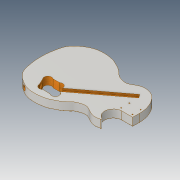
# Autodesk Inventor part: Corpo2
Saved by Autodesk Inventor 2016 (Build 200138000, 138)
## iProperties
Created: 2018-10-15
Part Number: Corpo2
Material: Generic
Document SubType Name: Modeling
Designer: Pedro Mendonça
Density: 1 g/cm^3
Appearance: Yellow Pine - Solid Stained Light Low Gloss
Author: Pedro Mendonça
Autodesk Inventor part; units mm, degrees
ref_plane "YZ Plane" through (0, 0, 0) normal (1, 0, 0) x (0, 1, 0)
ref_plane "XZ Plane" through (0, 0, 0) normal (0, 1, 0) x (-1, 0, 0)
ref_plane "XY Plane" through (0, 0, 0) normal (0, 0, 1) x (1, 0, 0)
sketch "Sketch1" plane through (0, 0, 0) normal (0, 0, 1) x (1, 0, 0)
  line L0 (0, 0) -> (0, -455) construction
  line L1 (0, -153) -> (-92, -153) construction
  line L2 (0, -435) -> (-103, -435) construction
  line L3 (0, -415) -> (-122, -415) construction
  line L4 (-0.0087, -394.9827) -> (-140.0087, -394.9827) construction
  line L5 (0, -375) -> (-151, -375) construction
  line L6 (0, -355) -> (-158, -355) construction
  line L7 (0, -335) -> (-160, -335) construction
  line L8 (0, -315) -> (-161, -315) construction
  line L9 (0, -295) -> (-158, -295) construction
  line L10 (0, -275) -> (-154, -275) construction
  line L11 (0, -255) -> (-145, -255) construction
  line L12 (0, -235) -> (-135, -235) construction
  line L13 (0, -215) -> (-120, -215) construction
  line L14 (0, -195) -> (-103, -195) construction
  line L15 (0, -175) -> (-95, -175) construction
  line L16 (0, -135) -> (-98, -135) construction
  line L17 (0, -115) -> (-109, -115) construction
  line L18 (0, -95) -> (-115, -95) construction
  line L19 (0, -75) -> (-114, -75) construction
  line L20 (0, -55) -> (-108, -55) construction
  line L21 (0, -35) -> (-93.9417, -35) construction
  line L22 (0, -15) -> (-65, -15) construction
  line L23 (0, -455) -> (-21.0472, -455.5046) construction
  line L24 (-159.5472, -351.6393) -> (-160.2622, -336.1037) construction
  line L25 (-64.2186, -11.8549) -> (-30.25, 0) construction
  line L26 (-30.25, 0) -> (0, 0) construction
  spline S0 degree 4 poles (0, -455) (-21.0472, -455.5046) (-39.9161, -452.9713) (-55.0288, -449.8264) (-72.5, -447.3805) (-90.9559, -441.7244) (-101.5897, -436.4609) (-110.5874, -430.5207) (-124.2149, -416.631) (-132.7759, -406.8471) (-140.8913, -395.5086) (-146.9896, -384.4071) (-152.044, -373.8933) (-155.7121, -363.9428) (-159.5472, -351.6393) (-160.2622, -336.1037) (-161.3959, -321.0408) (-160.7041, -310.0555) (-158.9541, -299.1238) (-157.4845, -291.3466) (-155.7121, -278.8181) (-152.3095, -270.0787) (-148.4765, -261.546) (-144.1012, -253.4714) (-138.9752, -242.9989) (-135, -233.5666) (-126.4423, -222.6445) (-115.9364, -209.2361) (-106.2015, -200.3968) (-100.5222, -191.8137) (-95.3552, -177.4658) (-92.8358, -167.4735) (-90.7434, -152.656) (-94.3304, -141.7669) (-99.2411, -132.3298) (-104.9533, -123.6353) (-111.1925, -111.3398) (-114.7925, -100.8201) (-115.9364, -86.2479) (-114.1418, -74.0378) (-111.6352, -63.1761) (-106.7365, -51.5397) (-99.6977, -40.3072) (-84.235, -25) (-64.2186, -11.8549) (-30.25, 0) (0, 0) knots 1 1 1 1 1 1.192103 1.235764 1.325453 1.466485 1.477925 1.676642 2 2.143283 3 3.486615 3.82198 4 5 6 6.816415 7 7.358575 8 8.561677 9 9.306621 10 10.059652 11 11.392225 12 12.736138 13 14 14.050123 15 15.249645 16 16.147201 17 17.733562 18 19 19.360293 20 20.169025 21 22 22 22 22 22
  line L27 (-99.6977, -40.3072) -> (-84.235, -25) construction
  line L28 (-84.235, -25) -> (-64.2186, -11.8549) construction
  line L29 (-114.1418, -74.0378) -> (-111.6352, -63.1761) construction
  line L30 (-111.6352, -63.1761) -> (-106.7365, -51.5397) construction
  line L31 (-106.7365, -51.5397) -> (-99.6977, -40.3072) construction
  line L32 (-114.7925, -100.8201) -> (-115.9364, -86.2479) construction
  line L33 (-115.9364, -86.2479) -> (-114.1418, -74.0378) construction
  line L34 (-104.9533, -123.6353) -> (-111.1925, -111.3398) construction
  line L35 (-111.1925, -111.3398) -> (-114.7925, -100.8201) construction
  line L36 (-94.3304, -141.7669) -> (-99.2411, -132.3298) construction
  line L37 (-99.2411, -132.3298) -> (-104.9533, -123.6353) construction
  line L38 (-95.3552, -177.4658) -> (-92.8358, -167.4735) construction
  line L39 (-92.8358, -167.4735) -> (-90.7434, -152.656) construction
  line L40 (-90.7434, -152.656) -> (-94.3304, -141.7669) construction
  line L41 (-106.2015, -200.3968) -> (-100.5222, -191.8137) construction
  line L42 (-100.5222, -191.8137) -> (-95.3552, -177.4658) construction
  line L43 (-126.4423, -222.6445) -> (-115.9364, -209.2361) construction
  line L44 (-115.9364, -209.2361) -> (-106.2015, -200.3968) construction
  line L45 (-138.9752, -242.9989) -> (-135, -233.5666) construction
  line L46 (-135, -233.5666) -> (-126.4423, -222.6445) construction
  line L47 (-148.4765, -261.546) -> (-144.1012, -253.4714) construction
  line L48 (-144.1012, -253.4714) -> (-138.9752, -242.9989) construction
  line L49 (-155.7121, -278.8181) -> (-152.3095, -270.0787) construction
  line L50 (-152.3095, -270.0787) -> (-148.4765, -261.546) construction
  line L51 (-158.9541, -299.1238) -> (-157.4845, -291.3466) construction
  line L52 (-157.4845, -291.3466) -> (-155.7121, -278.8181) construction
  line L53 (-160.2622, -336.1037) -> (-161.3959, -321.0408) construction
  line L54 (-161.3959, -321.0408) -> (-160.7041, -310.0555) construction
  line L55 (-160.7041, -310.0555) -> (-158.9541, -299.1238) construction
  line L56 (-146.9896, -384.4071) -> (-152.044, -373.8933) construction
  line L57 (-152.044, -373.8933) -> (-155.7121, -363.9428) construction
  line L58 (-155.7121, -363.9428) -> (-159.5472, -351.6393) construction
  line L59 (-132.7759, -406.8471) -> (-140.8913, -395.5086) construction
  line L60 (-140.8913, -395.5086) -> (-146.9896, -384.4071) construction
  line L61 (-124.2149, -416.631) -> (-132.7759, -406.8471) construction
  line L62 (-110.5874, -430.5207) -> (-124.2149, -416.631) construction
  line L63 (-90.9559, -441.7244) -> (-101.5897, -436.4609) construction
  line L64 (-101.5897, -436.4609) -> (-110.5874, -430.5207) construction
  line L65 (-21.0472, -455.5046) -> (-39.9161, -452.9713) construction
  line L66 (-39.9161, -452.9713) -> (-55.0288, -449.8264) construction
  line L67 (-55.0288, -449.8264) -> (-72.5, -447.3805) construction
  line L68 (-72.5, -447.3805) -> (-90.9559, -441.7244) construction
  line L69 (0, -455) -> (21.0472, -455.5046) construction
  line L70 (159.5472, -351.6393) -> (160.2622, -336.1037) construction
  line L71 (114.7925, -100.8201) -> (115.8966, -86.7554) construction
  line L72 (104.9533, -123.6353) -> (111.1925, -111.3398) construction
  line L73 (111.1925, -111.3398) -> (114.7925, -100.8201) construction
  line L74 (94.3304, -141.7669) -> (99.2411, -132.3298) construction
  line L75 (99.2411, -132.3298) -> (104.9533, -123.6353) construction
  line L76 (95.3552, -177.4658) -> (92.8358, -167.4735) construction
  line L77 (92.8358, -167.4735) -> (90.7434, -152.656) construction
  line L78 (90.7434, -152.656) -> (94.3304, -141.7669) construction
  line L79 (106.2015, -200.3968) -> (100.5222, -191.8137) construction
  line L80 (100.5222, -191.8137) -> (95.3552, -177.4658) construction
  line L81 (126.4423, -222.6445) -> (115.9364, -209.2361) construction
  line L82 (115.9364, -209.2361) -> (106.2015, -200.3968) construction
  line L83 (138.9752, -242.9989) -> (135, -233.5666) construction
  line L84 (135, -233.5666) -> (126.4423, -222.6445) construction
  line L85 (148.4765, -261.546) -> (144.1012, -253.4714) construction
  line L86 (144.1012, -253.4714) -> (138.9752, -242.9989) construction
  line L87 (155.7121, -278.8181) -> (152.3095, -270.0787) construction
  line L88 (152.3095, -270.0787) -> (148.4765, -261.546) construction
  line L89 (158.9541, -299.1238) -> (157.4845, -291.3466) construction
  line L90 (157.4845, -291.3466) -> (155.7121, -278.8181) construction
  line L91 (160.2622, -336.1037) -> (161.3959, -321.0408) construction
  line L92 (161.3959, -321.0408) -> (160.7041, -310.0555) construction
  line L93 (160.7041, -310.0555) -> (158.9541, -299.1238) construction
  line L94 (146.9896, -384.4071) -> (152.044, -373.8933) construction
  line L95 (152.044, -373.8933) -> (155.7121, -363.9428) construction
  line L96 (155.7121, -363.9428) -> (159.5472, -351.6393) construction
  line L97 (132.7759, -406.8471) -> (140.8913, -395.5086) construction
  line L98 (140.8913, -395.5086) -> (146.9896, -384.4071) construction
  line L99 (124.2149, -416.631) -> (132.7759, -406.8471) construction
  line L100 (110.5874, -430.5207) -> (124.2149, -416.631) construction
  line L101 (90.9559, -441.7244) -> (101.5897, -436.4609) construction
  line L102 (101.5897, -436.4609) -> (110.5874, -430.5207) construction
  line L103 (21.0472, -455.5046) -> (39.9161, -452.9713) construction
  line L104 (39.9161, -452.9713) -> (55.0288, -449.8264) construction
  line L105 (55.0288, -449.8264) -> (72.5, -447.3805) construction
  line L106 (72.5, -447.3805) -> (90.9559, -441.7244) construction
  line L107 (0, 0) -> (30, 0)
  line L108 (30, 0) -> (30, -50)
  line L109 (30, -50) -> (70, -50) construction
  arc A0 (30, -50) -> (106.5425, -66.2679) centre (70, -50) ccw
  arc A1 (112.1757, -66.6921) -> (106.5425, -66.2679) centre (109.2832, -67.488) ccw
  spline S1 degree 4 poles (0, -455) (21.0472, -455.5046) (39.9161, -452.9713) (55.0288, -449.8264) (72.5, -447.3805) (90.9559, -441.7244) (101.5897, -436.4609) (110.5874, -430.5207) (124.2149, -416.631) (132.7759, -406.8471) (140.8913, -395.5086) (146.9896, -384.4071) (152.044, -373.8933) (155.7121, -363.9428) (159.5472, -351.6393) (160.2622, -336.1037) (161.3959, -321.0408) (160.7041, -310.0555) (158.9541, -299.1238) (157.4845, -291.3466) (155.7121, -278.8181) (152.3095, -270.0787) (148.4765, -261.546) (144.1012, -253.4714) (138.9752, -242.9989) (135, -233.5666) (126.4423, -222.6445) (115.9364, -209.2361) (106.2015, -200.3968) (100.5222, -191.8137) (95.3552, -177.4658) (92.8358, -167.4735) (90.7434, -152.656) (94.3304, -141.7669) (99.2411, -132.3298) (104.9533, -123.6353) (111.1925, -111.3398) (114.7925, -100.8201) (115.8966, -86.7554) (114.5611, -76.9293) (113.4123, -71.1859) (112.1752, -66.6903) knots 1 1 1 1 1 1.192103 1.235764 1.325453 1.466485 1.477925 1.676642 2 2.143283 3 3.486615 3.82198 4 5 6 6.816415 7 7.358575 8 8.561677 9 9.306621 10 10.059652 11 11.392225 12 12.736138 13 14 14.050123 15 15.249645 16 16.147201 17 17.733562 18 18.900639 18.900639 18.900639 18.900639 18.900639
  line L110 (115.8966, -86.7554) -> (114.5611, -76.9293) construction
  line L111 (114.5611, -76.9293) -> (113.4123, -71.1859) construction
  line L112 (113.4123, -71.1859) -> (112.1752, -66.6903) construction
  dimension "d85" = 30
  dimension "d87" = 90
  dimension "d88" = 40
  dimension "d95" = 6
  constraints: 52 end point, 37 symmetric about line, 9 horizontal, 5 point on circle, 2 centre point, 1 coincident, 1 parallel, 1 perpendicular, 1 point on line, 1 tangent, 8 other
  measures "d85" distance of L26.end L107.end
  measures "d87" angle of L107 L108
  measures "d88" distance of L108.end L109.end
  measures "d95" diameter of A1
extrude "Extrusion1" add sketch "Sketch1" along normal blind 39
fillet "Fillet1" radius 2.9 7 edges at (112.1754, -66.6912, 19.5) (109.5075, -64.4964, 0) (61.6844, -89.1261, 0) (30, -25, 0) (140.5523, -246.0973, 0) (-120.2984, -214.9668, 0) (15, 0, 0)
sketch "Sketch2" plane through (0, 0, 0) normal (0, 0, -1) x (-1, 0, 0)
  line L0 (0, 0) -> (0, -12) construction
  line L1 (0, -12) -> (-19, -12) construction
  line L2 (0, -12) -> (19, -12) construction
  circle A0 centre (19, -12) radius 2.3
  circle A1 centre (-19, -12) radius 2.3
  line L3 (0, -12) -> (0, -64) construction
  line L4 (0, -52) -> (0, -64) construction
  line L5 (0, -64) -> (-19, -64) construction
  line L6 (0, -64) -> (19, -64) construction
  circle A2 centre (19, -64) radius 2.3
  circle A3 centre (-19, -64) radius 2.3
  dimension "d99" = 12
  dimension "d100" = 19
  dimension "d101" = 19
  dimension "d102" = 4.6
  dimension "d103" = 4.6
  dimension "d104" = 52
  dimension "d105" = 12
  dimension "d106" = 19
  dimension "d107" = 19
  dimension "d108" = 4.6
  dimension "d109" = 4.6
  constraints: 14 end point, 4 centre point, 4 coincident, 4 horizontal, 3 vertical
  measures "d99" distance of L0.start L0.end
  measures "d100" distance of L0.end L1.end
  measures "d101" distance of L0.end L2.end
  measures "d102" diameter of A0
  measures "d103" diameter of A1
  measures "d104" distance of L0.end L3.end
  measures "d105" distance of L4.start L4.end
  measures "d106" distance of L4.end L5.end
  measures "d107" distance of L4.end L6.end
  measures "d108" diameter of A2
  measures "d109" diameter of A3
extrude "Extrusion2" cut sketch "Sketch2" against normal through all
sketch "Sketch3" plane through (0, 0, 0) normal (0, 0, -1) x (-1, 0, 0)
  line L0 (0, 0) -> (0, -332) construction
  line L1 (0, -332) -> (-46, -332) construction
  line L2 (-46, -332) -> (-46, -297.4128)
  line L3 (-46, -332) -> (-46, -348.8838)
  line L4 (-85.3886, -374.4631) -> (-125.3109, -356.6885)
  line L5 (-141.9223, -331.1092) -> (-141.9223, -275.0602)
  line L6 (-60.3209, -272.9817) -> (-100.2431, -250.629)
  arc A0 (-85.3886, -374.4631) -> (-46, -348.8838) centre (-74, -348.8838) ccw
  arc A1 (-100.2431, -250.629) -> (-141.9223, -275.0602) centre (-113.9223, -275.0602) ccw
  arc A2 (-46, -297.4128) -> (-60.3209, -272.9817) centre (-74, -297.4128) ccw
  arc A3 (-141.9223, -331.1092) -> (-125.3109, -356.6885) centre (-113.9223, -331.1092) ccw
  point P0 (-46, -281)
  point P1 (-46, -392)
  point P2 (-141.9223, -349.2927)
  point P3 (-141.9223, -227.2927)
  dimension "d112" = 332
  dimension "d113" = 46
  dimension "d114" = 51
  dimension "d116" = 60
  dimension "d117" = 105
  dimension "d118" = 66
  dimension "d119" = 122
  dimension "d121" = 28
  dimension "d122" = 28
  dimension "d123" = 28
  constraints: 14 end point, 8 point on circle, 8 point on line, 8 tangent, 4 centre point, 4 vertical, 1 equal radius, 1 horizontal
  measures "d112" distance of L0.start L0.end
  measures "d113" distance of L0.end L1.end
  measures "d114" distance of L1.end point (-46, -281)
  measures "d116" distance of L1.end point (-46, -392)
  measures "d117" distance of point (-46, -392) point (-141.922, -349.293)
  measures "d118" angle of L3 L4
  measures "d119" distance of point (-141.922, -349.293) point (-141.922, -227.293)
  measures "d121" radius of A0
  measures "d122" radius of A1
  measures "d123" radius of A2
extrude "Extrusion3" cut sketch "Sketch3" against normal blind 3
sketch "Sketch4" plane through (0, 0, 3) normal (0, 0, -1) x (-1, 0, 0)
  arc A0 (-85.3886, -374.4631) -> (-46, -348.8838) centre (-74, -348.8838) ccw construction
  arc A1 (-141.9223, -331.1092) -> (-125.3109, -356.6885) centre (-113.9223, -331.1092) ccw construction
  arc A2 (-100.2431, -250.629) -> (-141.9223, -275.0602) centre (-113.9223, -275.0602) ccw construction
  arc A3 (-46, -297.4128) -> (-60.3209, -272.9817) centre (-74, -297.4128) ccw construction
  arc A4 (-86.5932, -361.0353) -> (-60.3209, -337.969) centre (-74, -348.8838) ccw
  arc A5 (-60.3209, -308.3276) -> (-71.7768, -280.0546) centre (-74, -297.4128) ccw
  arc A6 (-97.6917, -268.5166) -> (-127.0169, -286.6696) centre (-113.9223, -275.0602) ccw
  arc A7 (-127.0169, -319.4998) -> (-114.5261, -348.5988) centre (-113.9223, -331.1092) ccw
  line L0 (-85.3886, -374.4631) -> (-125.3109, -356.6885) construction
  line L1 (-100.2431, -250.629) -> (-60.3209, -272.9817) construction
  line L2 (-46, -297.4128) -> (-46, -348.8838) construction
  line L3 (-141.9223, -331.1092) -> (-141.9223, -275.0602) construction
  line L4 (-85.3886, -374.4631) -> (-125.3109, -356.6885) construction
  line L5 (-46, -297.4128) -> (-46, -348.8838) projected
  line L6 (-91.4726, -349.8633) -> (8.5274, -349.8633) construction
  line L7 (-60.3209, -337.969) -> (-60.3209, -308.3276)
  line L8 (-127.0169, -319.4998) -> (-127.0169, -286.6696)
  line L9 (-114.5261, -348.5988) -> (-86.5932, -361.0353)
  line L10 (-97.6917, -268.5166) -> (-71.7768, -280.0546)
  point P0 (0, 0)
  dimension "d126" = 35
  dimension "d128" = 35
  dimension "d129" = 35
  constraints: 18 end point, 16 point on circle, 8 centre point, 2 vertical, 1 coincident, 1 horizontal
  measures "d126" diameter of A4
  measures "d128" diameter of A6
  measures "d129" diameter of A7
extrude "Extrusion4" cut sketch "Sketch4" against normal through all
ref_plane "Work Plane1" through (86.5932, -361.0353, 3) normal (-0.809017, 0.5877853, 0) x (0, 0, 1)
sketch "Sketch5" plane through (86.5932, -361.0353, 3) normal (-0.809017, 0.5877853, 0) x (0, 0, 1)
  line L0 (0, 0) -> (0, 26.4799) construction
  line L1 (0, 26.4799) -> (36, 26.4799) construction
  line L2 (0, 0) -> (36, 0) construction
  line L3 (36, 26.4799) -> (36, 0) construction
  line L4 (18, 26.4799) -> (18, 0) construction
  line L5 (0, 0) -> (36, 0) projected
  line L6 (0, 13.2399) -> (36, 13.2399) construction
  circle A0 centre (18, 13.2399) radius 10.5
  point P0 (-3, 241.1855)
  dimension "d140" = 21
  constraints: 12 end point, 5 midpoint, 1 centre point
  measures "d140" diameter of A0
extrude "Extrusion5" cut sketch "Sketch5" against normal through all
ref_plane "Work Plane2" through (97.6917, -268.5166, 3) normal (0.601815, -0.7986355, 0) x (0, 0, 1)
sketch "Sketch6" plane through (97.6917, -268.5166, 3) normal (0.601815, -0.7986355, 0) x (0, 0, 1)
  line L0 (36, 27.6403) -> (36, 0) construction
  line L1 (0, 27.6403) -> (36, 27.6403) construction
  line L2 (0, 0) -> (0, 27.6403) construction
  line L3 (0, 0) -> (36, 0) construction
  line L4 (36, 13.8202) -> (36, 3.8202) construction
  line L5 (36, 3.8202) -> (26, 3.8202)
  line L6 (26, 3.8202) -> (26, 23.8202)
  line L7 (26, 23.8202) -> (36, 23.8202)
  line L8 (36, 23.8202) -> (36, 3.8202)
  point P0 (-3, -83.5772)
  dimension "d144" = 10
  dimension "d145" = 10
  dimension "d146" = 20
  constraints: 18 end point, 2 parallel, 1 horizontal, 1 midpoint, 1 perpendicular, 1 point on line
  measures "d144" distance of L4.start L4.end
  measures "d145" distance of L6.end L7.end
  measures "d146" distance of L5.end L6.end
extrude "Extrusion6" cut sketch "Sketch6" against normal blind 260
body "Solid1"
